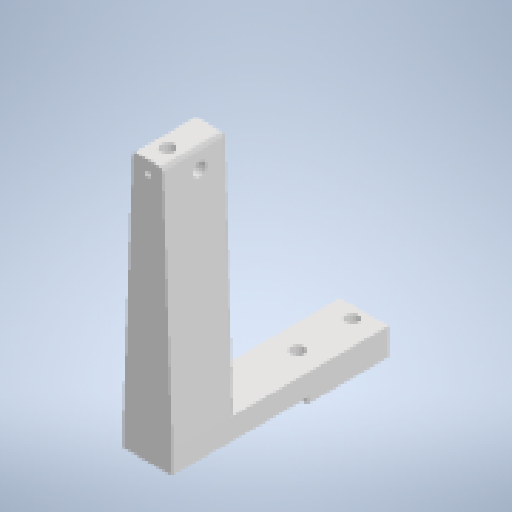
# Autodesk Inventor part: microstim_holder_bottom
Saved by Autodesk Inventor 2024 (Build 280153000, 153)
## iProperties
Created: 2023-05-03
Part Number: microstim_holder_bottom
Material: Generic
Document SubType Name: Modeling
Designer: Rober
Mass: 538.313 g
Surface Area: 676.575 cm^2
Volume: 538.313 cm^3
Density: 1 g/cm^3
Appearance: Default
Author: Rober
Autodesk Inventor part; units mm, degrees
ref_plane "YZ Plane" through (0, 0, 0) normal (1, 0, 0) x (0, 1, 0)
ref_plane "XZ Plane" through (0, 0, 0) normal (0, 1, 0) x (-1, 0, 0)
sketch "Sketch1" plane through (0, 0, 0) normal (0, 1, 0) x (-1, 0, 0)
  line L0 (3.05, -5.3255) -> (-3.05, -5.3255)
  line L1 (-3.05, -5.3255) -> (-3.05, 4.8245)
  line L2 (-3.05, 4.8245) -> (3.05, 4.8245)
  line L3 (3.05, 4.8245) -> (3.05, -5.3255)
  line L4 (0.925, 4.8245) -> (-0.925, 4.8245)
  line L5 (0.925, 4.8245) -> (0.925, -5.3255)
  line L6 (-0.925, 4.8245) -> (-0.925, -5.3255)
  circle A0 centre (0, 3.0245) radius 0.8
  circle A1 centre (0, -3.8255) radius 0.8
  line L7 (0, 4.8245) -> (0, -5.3255)
  line L8 (-3.05, 0) -> (3.05, 0)
  point P0 (0, 0)
  dimension "d13" = 6.1
  dimension "d44" = 1.85
  dimension "d45" = 2.125
  dimension "d46" = 1.6
  dimension "d47" = 1.6
  dimension "d128" = 6.85
  constraints: 18 end point, 9 point on line, 4 perpendicular, 3 midpoint, 2 centre point, 2 parallel, 1 horizontal
  measures "d13" distance of L0.start L0.end
  measures "d44" distance of L4.start L4.end
  measures "d45" distance from line of L3 L4.start
  measures "d46" diameter of A0
  measures "d47" diameter of A1
  measures "d128" distance of A0.centre A1.centre
extrude "Extrusion1" add sketch "Sketch1" along normal blind 3.4 contours L0 L5 L8 L3 | L0 L7 A1 L8 L5 | L8 L5 L2 L3 | L0 L6 L8 L7 A1 | L8 L7 A0 L2 L5 | L0 L1 L8 L6 | L8 L6 L2 L7 A0 | L8 L1 L2 L6
extrude "Extrusion6" add sketch "Sketch1" against normal blind 1 contours L0 L7 A1 L8 L5 | L0 L6 L8 L7 A1 | L8 L7 A0 L2 L5 | L8 L6 L2 L7 A0
sketch "Sketch13" plane through (-3.05, 3.4, 4.8245) normal (0, 0, 1) x (1, 0, 0)
  line L0 (0, 0) -> (0, -2.7)
  line L1 (0, -3.4) -> (0, 0) projected
  line L2 (0, -2.7) -> (6.1, -2.7)
  line L3 (6.1, -3.4) -> (6.1, 0) projected
  line L4 (6.1, 0) -> (6.1, -2.7)
  line L5 (0, 0) -> (6.1, 0)
  point P0 (3.05, -3.4)
  point P1 (6.1, -3.41)
  dimension "d56" = 2.7
  constraints: 8 end point, 3 perpendicular, 2 point on line
  measures "d56" distance of L0.start L0.end
extrude "Extrusion8" add sketch "Sketch13" along normal blind 17
sketch "Sketch17" plane through (-3.05, 3.4, 21.8245) normal (0, 0, 1) x (1, 0, 0)
  line L0 (6.1, 0) -> (0, 0) projected
  line L1 (6.1, 0) -> (19.567, 0) construction
  line L2 (16.968, 8.2706) -> (10.0894, 18.4685)
  line L3 (10.0894, 18.4685) -> (13.5713, 20.8172)
  line L4 (13.5713, 20.8172) -> (20.102, 11.1351)
  line L5 (20.102, 11.1351) -> (22.1374, 8.1174)
  line L6 (6.1, -3.4) -> (6.1, -2.7) projected
  line L7 (22.1374, 8.1174) -> (6.1, -2.7)
  line L8 (6.1, 0) -> (6.1, -2.7)
  line L9 (6.1, 0.94) -> (6.1, 0)
  line L10 (6.1, 0.94) -> (3.05, 0.94)
  line L11 (3.05, 0.94) -> (3.05, 0)
  line L12 (16.968, 8.2706) -> (6.1, 0.94)
  line L13 (6.1, 0.94) -> (7.7497, 0.94)
  point P0 (3.05, -3.4)
  dimension "d74" = 12.301
  dimension "d75" = 4.2
  dimension "d92" = 3.64
  dimension "d93" = 3.64
  dimension "d94" = 10.868
  dimension "d98" = 34
  constraints: 24 end point, 3 horizontal, 3 perpendicular, 2 point on line, 1 midpoint, 1 parallel, 1 vertical
  measures "d74" distance of L2.start L2.end
  measures "d75" distance of L2.end L3.end
  measures "d92" distance of L4.end L5.end
  measures "d93" distance of L6.end L9.start
  measures "d94" horizontal distance of L2.start L9.start
  measures "d98" angle of L13 L12
extrude "Extrusion12" [suppressed]
ref_plane "Work Plane3" through (-3.05, 3.4, 13.8245) normal (0, 0, 1) x (1, 0, 0)
sketch "Sketch29" plane through (-3.05, 3.4, 13.8245) normal (0, 0, 1) x (1, 0, 0)
  line L0 (3.85, -4.4) -> (2.25, -4.4) projected
  line L1 (3.05, -4.4) -> (3.05, 30.1)
  line L2 (4.95, 30.1) -> (3.05, 30.1)
  line L3 (3.05, 30.1) -> (1.15, 30.1)
  line L4 (6.1, -3.4) -> (6.1, 0) projected
  line L5 (4.95, 30.1) -> (6.1, 0)
  line L6 (0, -3.4) -> (0, 0) projected
  line L7 (1.15, 30.1) -> (0, 0)
  line L8 (0, 0) -> (6.1, 0)
  point P0 (3.05, -3.4)
  point P1 (3.0506, 28.6)
  dimension "d137" = 34.5
  dimension "d138" = 3.8
  constraints: 12 end point, 3 horizontal, 1 collinear, 1 midpoint, 1 vertical
  measures "d137" distance of L1.start L1.end
  measures "d138" distance of L2.start L3.end
extrude "Extrusion20" add sketch "Sketch29" along normal blind 8
fillet "Fillet6" radius 0.5 2 edges at (2.475, 18.45, 13.8245) (-2.475, 18.45, 13.8245)
sketch "Sketch14" plane through (0, 3.4, 0) normal (0, 1, 0) x (1, 0, 0)
  line L0 (3.05, 5.3255) -> (3.05, -21.8245) projected
  line L1 (3.05, -21.8245) -> (3.05, -13.8245)
  line L2 (3.05, -13.8245) -> (-3.05, -13.8245)
  line L3 (-3.05, 5.3255) -> (-3.05, -21.8245) projected
  line L4 (-3.05, -21.8245) -> (3.05, -21.8245)
  point P0 (0, 0)
  dimension "d59" = 8
  constraints: 6 end point, 2 point on line, 1 parallel, 1 perpendicular
  measures "d59" distance of L0.end L1.end
extrude "Extrusion9" [suppressed]
sketch "Sketch16" plane through (0, 35.4, 0) normal (0, 1, 0) x (1, 0, 0)
  circle A0 centre (-0.1175, -18.652) radius 1.5
  line L0 (1.9325, -20.707) -> (-1.9325, -20.707) projected
  line L1 (1.9325, -14.9419) -> (1.9325, -20.707) projected
  point P0 (0, 0)
  point P1 (0, -20.707)
  dimension "d67" = 3
  dimension "d68" = 2.055
  dimension "d69" = 2.05
  constraints: 1 centre point, 1 midpoint
  measures "d67" diameter of A0
  measures "d68" vertical distance of point (0, -20.707) A0.centre
  measures "d69" distance from line of L1 A0.centre
extrude "Extrusion11" [suppressed]
sketch "Sketch15" plane through (-3.05, 3.4, 21.8245) normal (0, 0, 1) x (1, 0, 0)
  line L0 (2.6762, 10.6502) -> (2.7739, 7.8519) construction
  line L1 (6.1, 0) -> (4.9825, 32) projected
  line L2 (1.6768, 10.6153) -> (1.7746, 7.817)
  line L3 (3.7733, 7.8868) -> (3.6756, 10.6851)
  arc A0 (3.6756, 10.6851) -> (1.6768, 10.6153) centre (2.6762, 10.6502) ccw
  arc A1 (1.7746, 7.817) -> (3.7733, 7.8868) centre (2.7739, 7.8519) ccw
  point P0 (3.05, -3.4)
  point P1 (2.7251, 9.251)
  dimension "d62" = 1.4
  dimension "d63" = 2
  dimension "d64" = 3.05
  constraints: 8 end point, 4 point on circle, 4 tangent, 2 centre point, 2 parallel, 1 midpoint
  measures "d62" distance of point (2.725, 9.251) L0.end
  measures "d63" diameter of A1
  measures "d64" distance from line of L1 point (2.725, 9.251)
extrude "Extrusion10" [suppressed]
sketch "Sketch20" plane through (10.5213, 24.2172, 21.8245) normal (-0.5591929, 0.8290376, 0) x (0.8290376, 0.5591929, 0)
  circle A0 centre (-2.15, 2.0494) radius 1.5
  line L0 (-4.2, 0) -> (-4.2, 4.1) projected
  line L1 (0, 0) -> (-4.2, 0) projected
  point P0 (-22.2646, 21.8245)
  point P1 (-2.1, 0)
  dimension "d82" = 3
  dimension "d83" = 2.05
  dimension "d84" = 2.05
  constraints: 1 centre point, 1 midpoint
  measures "d82" diameter of A0
  measures "d83" distance from line of L0 A0.centre
  measures "d84" distance of point (-2.1, 0) A0.centre
extrude "Extrusion14" [suppressed]
sketch "Sketch18" plane through (-3.05, 3.4, 21.8245) normal (0, 0, 1) x (1, 0, 0)
  line L0 (12.7441, 18.3775) -> (14.3099, 16.0562) construction
  line L1 (11.9151, 17.8183) -> (13.4808, 15.497)
  line L2 (15.1389, 16.6154) -> (13.5732, 18.9367)
  arc A0 (13.5732, 18.9367) -> (11.9151, 17.8183) centre (12.7441, 18.3775) ccw
  arc A1 (13.4808, 15.497) -> (15.1389, 16.6154) centre (14.3099, 16.0562) ccw
  line L3 (22.1374, 8.1174) -> (13.5713, 20.8172) projected
  line L4 (10.0894, 18.4685) -> (13.5713, 20.8172) projected
  point P0 (3.05, -3.4)
  point P1 (13.527, 17.2169)
  point P2 (12.1849, 19.2066)
  dimension "d78" = 1.4
  dimension "d79" = 2
  dimension "d89" = 0.56
  dimension "d90" = 2.05
  constraints: 8 end point, 5 point on circle, 4 tangent, 2 centre point, 2 parallel, 1 midpoint
  measures "d78" distance of point (13.527, 17.217) L0.end
  measures "d79" diameter of A1
  measures "d89" distance from line of L4 point (12.185, 19.207)
  measures "d90" distance from line of L3 point (13.527, 17.217)
extrude "Extrusion13" [suppressed]
sketch "Sketch21" plane through (13.7716, 15.5536, 19.7751) normal (-0.5591929, 0.8290376, 0) x (0.8290376, 0.5591929, 0)
  circle A0 centre (0, 0) radius 0.868
  point P0 (-20.1146, 19.7751)
  constraints: 1 centre point
extrude "Extrusion15" [suppressed]
mirror "Mirror3" [suppressed]
chamfer "Chamfer1" [suppressed]
fillet "Fillet1" [suppressed]
sketch "Sketch24" plane through (-3.05, 0, -5.3255) normal (-1, 0, 0) x (0, 0, 1)
  circle A0 centre (22.6257, 31.1455) radius 0.8
  point P0 (5.3255, 0)
  point P1 (27.15, 0.7)
  dimension "d109" = 1.6
  constraints: 1 centre point
  measures "d109" diameter of A0
extrude "Extrusion18" cut sketch "Sketch24" against normal through all
sketch "Sketch26" plane through (0, 35.4, 0) normal (0, 1, 0) x (1, 0, 0)
  circle A0 centre (0, -19.1945) radius 0.8
  point P0 (0, 0)
  dimension "d131" = 1.6
  constraints: 1 centre point
  measures "d131" diameter of A0
extrude "Extrusion19" [suppressed]
fillet "Fillet4" [suppressed]
sketch "Sketch31" plane through (-3.05, 3.4, 13.8245) normal (0, 0, -1) x (-1, 0, 0)
  line L0 (-3.05, -3.4) -> (-3.05, 28.5)
  circle A0 centre (-3.05, 28.5) radius 0.355
  dimension "d145" = 31.9
  dimension "d147" = 0.71
  constraints: 2 end point, 1 centre point, 1 coincident, 1 vertical
  measures "d145" distance of L0.start L0.end
  measures "d147" diameter of A0
extrude "Extrusion22" cut sketch "Sketch31" against normal through all
sketch "Sketch33" plane through (-1.9, 33.5, 21.8245) normal (0, 1, 0) x (1, 0, 0)
  line L0 (3.8, 0) -> (0, 0) projected
  line L1 (3.8, 7.5) -> (3.8, 0) projected
  line L2 (0, 7.5) -> (0, 0) projected
  circle A0 centre (1.9, 2.5) radius 0.8
  line L3 (1.9, 2.5) -> (3.8, 2.5)
  line L4 (1.9, 2.5) -> (0, 2.5)
  point P0 (1.9, 21.8245)
  dimension "d150" = 1.6
  dimension "d151" = 2.5
  constraints: 4 end point, 3 point on line, 1 centre point, 1 collinear, 1 perpendicular
  measures "d150" diameter of A0
  measures "d151" distance from line of L0 L3.start
extrude "Extrusion23" cut sketch "Sketch33" against normal blind 2 contours L3 L4 A0 | A0 L4 L3
fillet "Fillet7" radius 0.5 4 edges at (-1.9, 33.5, 18.0745) (1.7534, 33.5, 13.9709) (0, 33.5, 13.8245) (1.9, 33.5, 18.0745)
sketch "Sketch34" plane through (-3.05, 3.4, 13.8245) normal (0, 0, -1) x (-1, 0, 0)
  point P0 (-3.05, -3.4)
equation "\"d13\" = base_width"
equation "\"d45\" = -0.5 * d44 + 0.5 * d13"
equation "\"d4\" = base_length"
equation "\"base_width\" = 6.1"
equation "\"base_length\" = 3.4"
equation "\"base_screw_diameter\" = 1.5"
equation "\"base_screw_spacing_edge\" = 8.5"
equation "\"multi_angle\" = 34deg"
body "Solid1"
